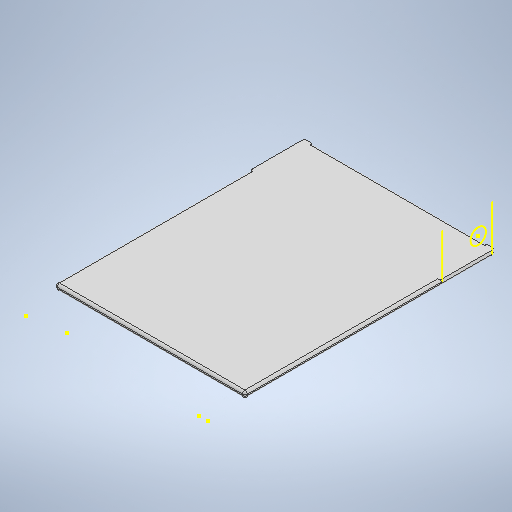
# Autodesk Inventor part: parte 1
Saved by Autodesk Inventor 2025.2 (Build 292293000, 293)
## iProperties
Created: 2025-02-16
Part Number: parte 1
Material: Generic
Document SubType Name: Modeling
Designer: maqmat
Density: 1 g/cm^3
Appearance: Default
Author: maqmat
Autodesk Inventor part; units mm, degrees
ref_plane "YZ Plane" through (0, 0, 0) normal (1, 0, 0) x (0, 1, 0)
ref_plane "XZ Plane" through (0, 0, 0) normal (0, 1, 0) x (-1, 0, 0)
ref_plane "XY Plane" through (0, 0, 0) normal (0, 0, 1) x (1, 0, 0)
sketch "Sketch1" plane through (0, 0, 0) normal (0, 1, 0) x (-1, 0, 0)
  line L0 (41.5241, -31.4619) -> (-118.4759, -31.4619)
  line L1 (-118.4759, -31.4619) -> (-118.4759, -241.4619)
  line L2 (-118.4759, -241.4619) -> (41.5241, -241.4619)
  line L3 (41.5241, -241.4619) -> (41.5241, -31.4619)
  line L4 (-118.4759, -241.4619) -> (-109.4759, -241.4619)
  line L5 (-118.4759, -195.4619) -> (-118.4759, -241.4619)
  line L6 (41.5241, -31.4619) -> (32.5241, -31.4619)
  line L7 (41.5241, -77.4619) -> (41.5241, -31.4619)
  line L8 (41.5241, -31.4619) -> (41.5241, -77.4619)
  line L9 (-118.4759, -195.4619) -> (-118.4759, -241.4619)
  line L10 (41.5241, -195.657) -> (41.5241, -77.4619)
  line L11 (-118.4759, -195.4619) -> (-118.4759, -241.4619)
  line L12 (41.5241, -195.657) -> (41.5241, -77.4619)
  line L13 (-118.4759, -241.4619) -> (-111.4759, -241.4619)
  line L14 (-118.4759, -195.4619) -> (-118.4759, -241.4619)
  line L15 (41.5241, -77.4619) -> (41.5241, -195.657)
  line L16 (-118.4759, -241.4619) -> (-111.4759, -241.4619)
  line L17 (-111.4759, -241.4619) -> (-111.4759, -195.4619)
  line L18 (-111.4759, -195.4619) -> (-118.4759, -195.4619)
  line L19 (-118.4759, -195.4619) -> (-118.4759, -241.4619)
  line L20 (41.5241, -195.657) -> (34.5241, -195.657)
  line L21 (34.5241, -195.657) -> (34.5241, -241.657)
  line L22 (41.5241, -241.657) -> (41.5241, -195.657)
  point P0 (0, 0)
  point P1 (34.5241, -31.4619)
  point P2 (34.5241, -241.4619)
  dimension "d0" = 160
  dimension "d1" = 210
  dimension "d14" = 7
  dimension "d15" = 46
  dimension "d16" = 7
  dimension "d17" = 46
  constraints: 46 end point, 6 horizontal, 5 parallel, 3 perpendicular, 1 collinear, 1 vertical
  measures "d0" distance of L2.end L1.end
  measures "d1" distance of L1.end L0.end
  measures "d14" distance of L18.end L17.end
  measures "d15" distance of L17.end L16.end
  measures "d16" distance of L22.start L21.end
  measures "d17" distance of L21.end L20.end
extrude "Extrusion3" add sketch "Sketch1" along normal blind 5
sketch "Sketch2" plane through (0, 5, 0) normal (0, 1, 0) x (1, 0, 0)
  point P0 (0, 0)
extrude "Extrusion4" add sketch "Sketch1" along normal blind 42 contours L3 L2 L21 L20 | L18 L17 L2 L1
sketch "Sketch3" plane through (-34.5241, 5, -77.4619) normal (1, 0, 0) x (0, 0, -1)
  point P0 (-77.4619, -5)
sketch "Sketch5" plane through (111.4759, 5, -195.4619) normal (-1, 0, 0) x (0, 0, 1)
  point P0 (195.4619, -5)
sketch "Sketch6" plane through (111.4759, 5, -195.4619) normal (-1, 0, 0) x (0, 0, 1)
  line L0 (-46, 0) -> (-46, 37) projected
  line L1 (0, 0) -> (0, 37) projected
  circle A0 centre (-32.1829, 16) radius 6.5
  line L2 (-46, 18.5) -> (-39.25, 18.5)
  point P0 (195.4619, -5)
  dimension "d72" = 6.75
  constraints: 2 end point, 1 centre point, 1 midpoint
  measures "d72" distance of L2.start L2.end
extrude "Extrusion6" cut sketch "Sketch6" against normal blind 10
sketch "Sketch8" plane through (111.4759, 5, -195.4619) normal (-1, 0, 0) x (0, 0, 1)
  line L0 (0, 0) -> (0, 37) projected
  line L1 (0, 18.5) -> (-3, 18.5)
  line L2 (-0.1952, 0) -> (164, 0) projected
  line L3 (0, 37) -> (-46, 37) projected
  line L4 (0, 32) -> (0, 27)
  line L5 (-46, -5) -> (-46, 37) projected
  line L6 (-46, 37) -> (-43, 37)
  circle A0 centre (-41.7831, 25.7499) radius 1.5
  circle A1 centre (-41.7831, 6.1836) radius 1.5
  circle A2 centre (-4.2217, 6.1836) radius 1.5
  circle A3 centre (-4.2217, 25.7499) radius 1.5
  point P0 (195.4619, -5)
  point P1 (-46, 0)
  point P2 (118, 0)
  dimension "d47" = 3
  constraints: 6 end point, 4 centre point, 2 horizontal, 1 midpoint, 1 vertical
  measures "d47" diameter of A3
extrude "Extrusion7" cut sketch "Sketch8" against normal blind 10 contours A2 | A3
extrude "Extrusion8" cut sketch "Sketch8" against normal blind 10 contours A0 | A1 | A2
thread "Thread5" size "M3x0.5" class "6H" standard "ANSI Metric M Profile" full length
thread "Thread6" size "M3x0.5" class "6H" standard "ANSI Metric M Profile" full length
thread "Thread7" size "M3x0.5" class "6H" standard "ANSI Metric M Profile" full length
thread "Thread8" size "M3x0.5" class "6H" standard "ANSI Metric M Profile" full length
fillet "Fillet1" radius 2 20 edges at (-41.5241, 2.5, -31.4619) (38.4759, 5, -31.4619) (118.4759, 2.5, -31.4619) (38.4759, 0, -31.4619) (118.4759, 0, -136.4619) (118.4759, 5, -113.4619) (118.4759, 23.5, -195.4619) (111.4759, 23.5, -195.4619) (118.4759, 42, -218.4619) (114.9759, 42, -195.4619) (118.4759, 21, -241.4619) (-34.5241, 42, -218.5595) (111.4759, 23.5, -241.4619) (38.4759, 5, -241.4619) (38.4759, 0, -241.4619) (111.4759, 42, -218.4619) (-41.5241, 42, -218.5595) (-41.5241, 5, -113.5595) (-41.5241, 21, -241.4619) (-41.5241, 0, -136.4619)
sketch "Sketch9" plane through (118.4759, 2, -239.4619) normal (1, 0, 0) x (0, 0, -1)
  circle A0 centre (-11.8171, 19) radius 6.5 projected
  line L0 (-42, 1) -> (-42, 38) projected
  line L1 (0, 38) -> (0, 0) projected
  point P0 (-239.4619, -2)
sketch "Sketch10" plane through (-34.5241, 37.0758, -195.5564) normal (1, 0, 0) x (0, 0, 1)
  line L0 (-46, 0) -> (-46, 37)
  line L1 (0, 0) -> (0, 37)
  circle A0 centre (-32.1829, 16) radius 6.5
  line L2 (-46, 18.5) -> (-39.25, 18.5)
  point P0 (195.4619, -5)
  dimension "d73" = 6.75
  constraints: 6 end point, 1 centre point, 1 midpoint
  measures "d73" distance of L2.start L2.end
extrude "Extrusion10" cut sketch "Sketch10" against normal blind 10
sketch "Sketch11" plane through (-41.5241, 5.1313, -195.4287) normal (-1, 0, 0) x (0, 0, 1)
  line L0 (0, 0) -> (0, 37)
  line L1 (0, 18.5) -> (-3, 18.5)
  line L2 (-0.1952, 0) -> (164, 0)
  line L3 (0, 37) -> (-46, 37)
  line L4 (0, 32) -> (0, 27)
  line L5 (-46, -5) -> (-46, 37)
  line L6 (-46, 37) -> (-43, 37)
  circle A0 centre (-41.7831, 25.7499) radius 1.5
  circle A1 centre (-41.7831, 6.1836) radius 1.5
  circle A2 centre (-4.2217, 6.1836) radius 1.5
  circle A3 centre (-4.2217, 25.7499) radius 1.5
  point P0 (195.4619, -5)
  point P1 (-46, 0)
  point P2 (118, 0)
  dimension "d77" = 3
  constraints: 14 end point, 4 centre point, 2 horizontal, 1 midpoint, 1 vertical
  measures "d77" diameter of A3
extrude "Extrusion11" cut sketch "Sketch11" against normal blind 10 contours A0 | A1 | A2
sketch "Sketch12" plane through (-41.5241, 5.0284, -195.4263) normal (-1, 0, 0) x (0, 0, 1)
  line L0 (0, 0) -> (0, 37)
  line L1 (0, 18.5) -> (-3, 18.5)
  line L2 (-0.1952, 0) -> (164, 0)
  line L3 (0, 37) -> (-46, 37)
  line L4 (0, 32) -> (0, 27)
  line L5 (-46, -5) -> (-46, 37)
  line L6 (-46, 37) -> (-43, 37)
  circle A0 centre (-41.7831, 25.7499) radius 1.5
  circle A1 centre (-41.7831, 6.1836) radius 1.5
  circle A2 centre (-4.2217, 6.1836) radius 1.5
  circle A3 centre (-4.2217, 25.7499) radius 1.5
  point P0 (195.4619, -5)
  point P1 (-46, 0)
  point P2 (118, 0)
  dimension "d81" = 3
  constraints: 14 end point, 4 centre point, 2 horizontal, 1 midpoint, 1 vertical
  measures "d81" diameter of A3
extrude "Extrusion12" cut sketch "Sketch12" against normal blind 10 contours A2 | A3
thread "Thread9" size "M3x0.5" class "6H" standard "ANSI Metric M Profile" full length
thread "Thread10" size "M3x0.5" class "6H" standard "ANSI Metric M Profile" full length
thread "Thread11" size "M3x0.5" class "6H" standard "ANSI Metric M Profile" full length
thread "Thread12" size "M3x0.5" class "6H" standard "ANSI Metric M Profile" full length
thread "Thread13" size "M3x0.5" class "6H" standard "ANSI Metric M Profile" full length
thread "Thread14" size "M3x0.5" class "6H" standard "ANSI Metric M Profile" full length
fillet "Fillet2" radius 2 4 edges at (-35.1099, 41.4142, -241.4619) (-38.0241, 42, -241.4619) (-40.9383, 41.4142, -240.8761) (-34.5241, 21.5, -241.4619)
fillet "Fillet3" radius 2 5 edges at (-35.1099, 41.4142, -195.657) (-38.0241, 42, -195.657) (-40.9383, 41.4142, -195.657) (-41.5241, 21.5, -195.657) (-34.5241, 22.5, -195.657)
sketch "Sketch13" plane through (118.4759, 2, -239.4619) normal (1, 0, 0) x (0, 0, -1)
  line L0 (-44, 3) -> (-206, 3) projected
  line L1 (-45.1841, 3) -> (7.708, 3)
  line L2 (7.708, 3) -> (7.708, 40)
  line L3 (7.708, 40) -> (-45.1841, 40)
  line L4 (-45.1841, 40) -> (-45.1841, 3)
  point P0 (-239.4619, -2)
  constraints: 8 end point, 2 parallel, 1 horizontal, 1 perpendicular, 1 point on line
extrude "Extrusion13" cut sketch "Sketch13" against normal blind 1111111
body "Solid2"
